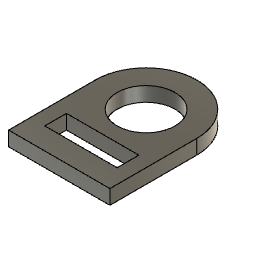
Exercise_1 (Autodesk Fusion 360 design; units mm, degrees)
Autodesk Fusion 360 part; units mm, degrees
sketch "Sketch1" plane through (0, 0, 0) normal (0, 1, 0) x (1, 0, 0)
  line L0 (0, 0) -> (70, 0)
  line L1 (0, 0) -> (0, -60)
  line L2 (70, 0) -> (70, -60)
  arc A0 (0, -60) -> (70, -60) centre (35, -60) ccw
  line L3 (10, -15) -> (60, -15)
  line L4 (10, -30) -> (10, -15)
  arc A1 (15, -60) -> (55, -60) centre (35, -60) ccw
  circle A2 centre (35, -60) radius 20
  line L5 (10, -30) -> (60, -30)
  line L6 (60, -30) -> (60, -15)
  dimension "d1" = 70
  dimension "d8" = 35
  dimension "d12" = 20
  dimension "d13" = 10
  dimension "d14" = 15
  dimension "d17" = 60
  dimension "d18" = 50
  dimension "d19" = 15
  constraint coincident L0.start L1.start
  constraint horizontal L0
  constraint perpendicular L0 L1
  constraint perpendicular L0 L2
  constraint tangent L1 A0
  constraint concentric A0 A1
  constraint perpendicular L3 L4
  constraint concentric A0 A2
  constraint coincident A1.start A2
  constraint perpendicular L4 L5
  constraint perpendicular L3 L6
  measures "d1" distance of L0.start L0.end
  measures "d8" radius of A0
  measures "d12" radius of A1
  measures "d13" distance of L1 L4
  measures "d14" distance of L0 L3
  measures "d17" distance of L0.start L1.end
  measures "d18" distance of L4.start L5.end
  measures "d19" distance of L3.end L5.end
extrude "Extrude1" add sketch "Sketch1" along normal blind 10
move_body "Move1" bodies 1 to x (1, 0, 0) y (0, 0, -1) z (0, 1, 0) at (22.9515, -60.0594, 30.5019)
move_body "Move2" bodies 1 to x (1, 0, 0) y (0, 1, 0) z (0, 0, 1) at (-15.563, 6.3564, -20.156)
